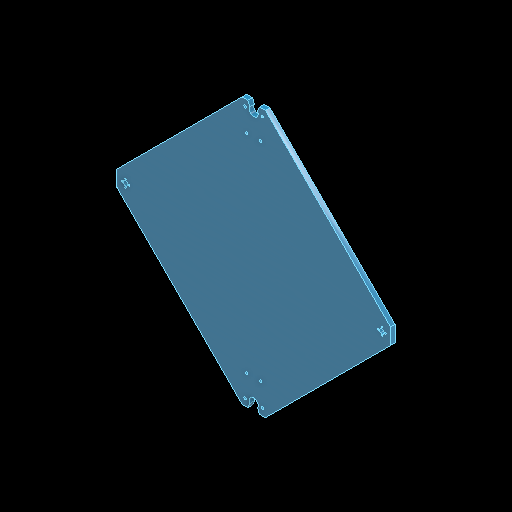
# Autodesk Inventor part: z_plate
Saved by Autodesk Inventor 2026.1 (Build 301233000, 233)
## iProperties
Created: 2025-09-21
Part Number: z_plate
Material: Aluminum 6061
Document SubType Name: Modeling
Designer: drago
Density: 2.7 g/cm^3
Appearance: Sky Blue Dark
Author: drago
Autodesk Inventor part; units mm, degrees
ref_plane "YZ Plane" through (0, 0, 0) normal (1, 0, 0) x (0, 1, 0)
ref_plane "XZ Plane" through (0, 0, 0) normal (0, 1, 0) x (-1, 0, 0)
ref_plane "XY Plane" through (0, 0, 0) normal (0, 0, 1) x (1, 0, 0)
sketch "Sketch2" plane through (0, 0, 0) normal (0, 0, 1) x (1, 0, 0)
  circle A0 centre (0, 277.5) radius 8 construction
  circle A1 centre (0, 277.5) radius 10
  circle A2 centre (0, 277.5) radius 10.5 construction
  line L0 (25, 287.5) -> (-25, 287.5) construction
  line L1 (-25, 287.5) -> (-25, 222.5) construction
  line L2 (-25, 222.5) -> (25, 222.5) construction
  line L3 (25, 222.5) -> (25, 287.5) construction
  circle A3 centre (15, 228.5) radius 2.7
  circle A4 centre (-15, 228.5) radius 2.7
  circle A5 centre (-19, 277.5) radius 2.7
  circle A6 centre (19, 277.5) radius 2.7
  circle A7 centre (0, -277.5) radius 8 construction
  circle A8 centre (0, -277.5) radius 10
  circle A9 centre (0, -277.5) radius 10.5 construction
  line L4 (25, -287.5) -> (-25, -287.5) construction
  line L5 (-25, -287.5) -> (-25, -222.5) construction
  line L6 (-25, -222.5) -> (25, -222.5) construction
  line L7 (25, -222.5) -> (25, -287.5) construction
  circle A10 centre (-15, -228.5) radius 2.7
  circle A11 centre (15, -228.5) radius 2.7
  circle A12 centre (-19, -277.5) radius 2.7
  circle A13 centre (19, -277.5) radius 2.7
  line L8 (10.5, -277.5) -> (10.5, -287.5) construction
  line L9 (-10.5, -277.5) -> (-10.5, -287.5) construction
  line L10 (10.5, 277.5) -> (10.5, 287.5) construction
  line L11 (-10.5, 277.5) -> (-10.5, 287.5) construction
  circle A14 centre (281.7, 0) radius 5.25
  circle A15 centre (289.7, 0) radius 1.6
  circle A16 centre (281.7, 8) radius 1.6
  circle A17 centre (273.7, 0) radius 1.6
  circle A18 centre (281.7, -8) radius 1.6
  circle A19 centre (-281.7, 0) radius 5.25
  circle A20 centre (-289.7, 0) radius 1.6
  circle A21 centre (-281.7, -8) radius 1.6
  circle A22 centre (-273.7, 0) radius 1.6
  circle A23 centre (-281.7, 8) radius 1.6
  line L12 (0, -318.1981) -> (318.1981, 0)
  line L13 (318.1981, 0) -> (0, 318.1981)
  line L14 (0, 318.1981) -> (-318.1981, 0)
  line L15 (-318.1981, 0) -> (0, -318.1981)
  line L16 (0, -318.1981) -> (0, 318.1981) construction
  line L17 (318.1981, 0) -> (-318.1981, 0) construction
  line L18 (0, -318.1981) -> (450, -318.1981) construction
  line L19 (300.5, 17.6981) -> (300.5, -17.6981)
  line L20 (-300.5, 17.6981) -> (-300.5, -17.6981)
  line L21 (-20.6981, 297.5) -> (20.6981, 297.5) construction
  line L22 (-25.6981, 292.5) -> (25.6981, 292.5)
  line L23 (-20.6981, -297.5) -> (20.6981, -297.5) construction
  line L24 (-25.6981, -292.5) -> (25.6981, -292.5)
  line L25 (-9.5, 297.5) -> (-3.976, 284.442) construction
  line L26 (9.5, 297.5) -> (3.976, 284.442) construction
  line L27 (-14.929, 297.5) -> (-8.6158, 282.5763)
  line L28 (14.929, 297.5) -> (8.6158, 282.5763)
  line L29 (-9.5, -297.5) -> (-3.976, -284.442) construction
  line L30 (9.5, -297.5) -> (3.976, -284.442) construction
  line L31 (14.929, -297.5) -> (8.6158, -282.5763)
  line L32 (-14.929, -297.5) -> (-8.6158, -282.5763)
  point P0 (0, 0)
  point P1 (-12.8138, -292.5)
  point P2 (12.8138, -292.5)
  point P3 (12.8138, 292.5)
  point P4 (-12.8138, 292.5)
  point P5 (300.5, 292.5)
  point P6 (300.5, -292.5)
  point P7 (-300.5, -292.5)
  point P8 (-300.5, 292.5)
  dimension "d256" = 16
  dimension "d257" = 0
  dimension "d258" = 277.5
  dimension "d259" = 20
  dimension "d260" = 21
  dimension "d261" = 50
  dimension "d262" = 10
  dimension "d263" = 65
  dimension "d265" = 50
  dimension "d266" = 25
  dimension "d267" = 5.4
  dimension "d268" = 5.4
  dimension "d269" = 5.4
  dimension "d270" = 5.4
  dimension "d271" = 6
  dimension "d272" = 10
  dimension "d273" = 6
  dimension "d274" = 10
  dimension "d275" = 6
  dimension "d276" = 10
  dimension "d277" = 6
  dimension "d278" = 10
  dimension "d279" = 0
  dimension "d280" = 277.5
  dimension "d281" = 20
  dimension "d282" = 16
  dimension "d283" = 21
  dimension "d284" = 50
  dimension "d285" = 10
  dimension "d286" = 65
  dimension "d287" = 25
  dimension "d288" = 5.4
  dimension "d289" = 5.4
  dimension "d290" = 5.4
  dimension "d291" = 5.4
  dimension "d292" = 6
  dimension "d293" = 10
  dimension "d294" = 6
  dimension "d295" = 10
  dimension "d296" = 10
  dimension "d297" = 6
  dimension "d298" = 10
  dimension "d299" = 6
  dimension "d300" = 10.5
  dimension "d301" = 0
  dimension "d302" = 281.7
  dimension "d303" = 3.2
  dimension "d304" = 0
  dimension "d305" = 8
  dimension "d308" = 360
  dimension "d310" = 10.5
  dimension "d311" = 0
  dimension "d312" = 281.7
  dimension "d313" = 3.2
  dimension "d314" = 0
  dimension "d315" = 8
  dimension "d318" = 360
  dimension "d320" = 450
  dimension "d321" = 45
  dimension "d322" = 450
  dimension "d323" = 18.8
  dimension "d324" = 18.8
  dimension "d325" = 20
  dimension "d326" = 15
  constraints: 66 end point, 28 point on line, 24 centre point, 12 point on circle, 6 horizontal, 5 perpendicular, 4 coincident, 4 parallel, 4 vertical, 2 midpoint, 2 tangent, 1 equal length, 19 other
  measures "d256" diameter of A0
  measures "d257" horizontal distance of point (0, 0) A0.centre
  measures "d258" distance of point (0, 0) A0.centre
  measures "d259" diameter of A1
  measures "d260" diameter of A2
  measures "d261" distance of L0.start L0.end
  measures "d262" distance from line of A2.centre L0
  measures "d263" distance of L0.end L1.end
  measures "d265" distance of L1.end L2.end
  measures "d266" distance from line of A2.centre L1
  measures "d267" diameter of A3
  measures "d268" diameter of A4
  measures "d269" diameter of A5
  measures "d270" diameter of A6
  measures "d271" distance from line of L2 A3.centre
  measures "d272" distance from line of L3 A3.centre
  measures "d273" distance from line of L2 A4.centre
  measures "d274" distance from line of L1 A4.centre
  measures "d275" distance from line of L3 A6.centre
  measures "d276" distance from line of L0 A6.centre
  measures "d277" distance from line of L1 A5.centre
  measures "d278" distance from line of L0 A5.centre
  measures "d279" horizontal distance of point (0, 0) A8.centre
  measures "d280" distance of point (0, 0) A8.centre
  measures "d281" diameter of A8
  measures "d282" diameter of A7
  measures "d283" diameter of A9
  measures "d284" distance of L4.start L4.end
  measures "d285" distance from line of L4 A8.centre
  measures "d286" distance of L4.end L5.end
  measures "d287" distance from line of A8.centre L5
  measures "d288" diameter of A10
  measures "d289" diameter of A11
  measures "d290" diameter of A12
  measures "d291" diameter of A13
  measures "d292" distance from line of L6 A10.centre
  measures "d293" distance from line of L5 A10.centre
  measures "d294" distance from line of L6 A11.centre
  measures "d295" distance from line of L7 A11.centre
  measures "d296" distance from line of L4 A12.centre
  measures "d297" distance from line of L5 A12.centre
  measures "d298" distance from line of L4 A13.centre
  measures "d299" distance from line of L7 A13.centre
  measures "d300" diameter of A14
  measures "d301" vertical distance of A14.centre point (0, 0)
  measures "d302" distance of point (0, 0) A14.centre
  measures "d303" diameter of A15
  measures "d304" vertical distance of A14.centre A15.centre
  measures "d305" distance of A14.centre A15.centre
  measures "d310" diameter of A19
  measures "d311" vertical distance of point (0, 0) A19.centre
  measures "d312" distance of point (0, 0) A19.centre
  measures "d313" diameter of A20
  measures "d314" vertical distance of A19.centre A20.centre
  measures "d315" distance of A19.centre A20.centre
  measures "d320" distance of L12.start L12.end
  measures "d321" angle of L18 L12
  measures "d322" distance of L13.end L12.end
  measures "d323" distance from line of L19 A14.centre
  measures "d324" distance from line of A19.centre L20
  measures "d325" distance from line of A1.centre L21
  measures "d326" distance from line of A1.centre L22
extrude "Extrusion11" add sketch "Sketch2" against normal blind 10 contours A1 L28 L22 L13 L19 L12 L24 L31 A8 L32 L15 L20 L14 L27
equation "\"diag_dist_rails\" = 555"
equation "\"diag_dist_leadscrews\" = 563.4"
equation "\"diam_leadscrew_hole\" = 10.5"
equation "\"delta\" = 5"
equation "\"phi\" = 67.07deg"
equation "\"D\" = 9.5"
body "Solid10"
